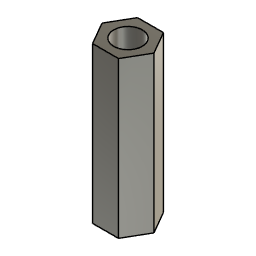
Distance_M2_12mm (Autodesk Fusion 360 design; units mm, degrees)
part number: 2025-04-02-17-14-34-310
Autodesk Fusion 360 part; units mm, degrees
sketch "Szkic1" plane through (0, 0, 0) normal (0, 0, 1) x (1, 0, 0)
  line L0 (0, 0) -> (2, 0)
  line L1 (2, 0) -> (3, 1.7321)
  line L2 (3, 1.7321) -> (2, 3.4641)
  line L3 (2, 3.4641) -> (0, 3.4641)
  line L4 (0, 3.4641) -> (-1, 1.7321)
  line L5 (-1, 1.7321) -> (0, 0)
  point P0 (1, 1.7321)
  constraint coincident L0.start L5.end
extrude "Wyciągnięcie proste1" add sketch "Szkic1" along normal blind 12
sketch "Szkic2" plane through (0, 0, 12) normal (0, 0, 1) x (-1, 0, 0)
  line L0 (1, -1.7321) -> (0, 0)
  line L1 (0, 0) -> (-2, 0)
  line L2 (-2, 0) -> (-3, -1.7321)
  line L3 (-3, -1.7321) -> (-2, -3.4641)
  line L4 (-2, -3.4641) -> (0, -3.4641)
  line L5 (0, -3.4641) -> (1, -1.7321)
  line L6 (1, -1.7321) -> (0, 0)
  line L7 (0, 0) -> (-2, 0)
  line L8 (-2, 0) -> (-3, -1.7321)
  line L9 (-3, -1.7321) -> (-2, -3.4641)
  line L10 (-2, -3.4641) -> (0, -3.4641)
  line L11 (0, -3.4641) -> (1, -1.7321)
  line L12 (1, -1.7321) -> (-3, -1.7321)
  line L13 (-2, -3.4641) -> (0, 0)
  circle A0 centre (-1, -1.7321) radius 1.1
  dimension "d3" = 2.2
  constraint coincident L0.start L5.end
  constraint horizontal L12
  constraint midpoint L13 A0.centre
  measures "d3" diameter of A0
hole "Otwór1" at (1, 1.7321, 12) direction (0, 0, -1) diameter 2.2 end through all
